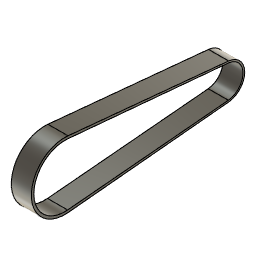
同步带2 v2 (Autodesk Fusion 360 design; units mm, degrees)
Autodesk Fusion 360 part; units mm, degrees
sketch "草图1" plane through (0, 0, 0) normal (1, 0, 0) x (0, 1, 0)
  circle A0 centre (0, 0) radius 9.25
  circle A1 centre (0, 0) radius 10
  line L0 (0, 0) -> (48.5, 0)
  circle A2 centre (48.5, 0) radius 4.85
  circle A3 centre (48.5, 0) radius 5.35
  line L1 (49.0129, 5.3254) -> (0.9588, 9.9539)
  line L2 (49.0129, -5.3254) -> (0.9588, -9.9539)
  line L3 (0.8392, -9.2119) -> (48.94, -4.83)
  line L4 (0.8392, 9.2119) -> (48.94, 4.83)
  dimension "d1" = 18.5
  dimension "d2" = 20
  dimension "d3" = 48.5
  dimension "d4" = 9.7
  dimension "d5" = 10.7
  constraint coincident A0.centre A1.centre
  constraint concentric A0 A1
  constraint horizontal L0
  constraint coincident L0.end A2.centre
  constraint concentric A2 A3
  constraint coincident A3 L1.start
  constraint coincident A1 L1.end
  constraint tangent A1 L1
  constraint tangent A3 L1
  constraint symmetric L0 L1.start L2.start
  constraint symmetric L0 L1.end L2.end
  constraint coincident A0 L3.start
  constraint coincident A2 L3.end
  constraint tangent A2 L3
  constraint tangent A0 L3
  constraint symmetric L0 L3.start L4.start
  constraint symmetric L0 L3.end L4.end
  measures "d1" diameter of A0
  measures "d2" diameter of A1
  measures "d3" distance of A0.centre L0.end
  measures "d4" diameter of A2
  measures "d5" diameter of A3
extrude "拉伸1" add sketch "草图1" along normal blind 6 contours A0 A1 L3 L4 | A1 A3 L1 L4 | A1 A3 L2 L3 | A2 A3 L3 L4
